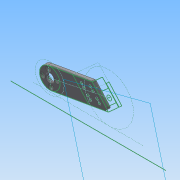
# Autodesk Inventor part: Motor Mount
Saved by Autodesk Inventor 2014 SP2 (Build 180246200, 246)
## iProperties
Created: 2014-05-16
Part Number: Motor Mount
Material: Generic
Document SubType Name: Modeling
Designer: dliu
Density: 1 g/cm^3
Appearance: Default
Author: dliu
Autodesk Inventor part; units mm, degrees
ref_plane "YZ Plane" through (0, 0, 0) normal (1, 0, 0) x (0, 1, 0)
ref_plane "XZ Plane" through (0, 0, 0) normal (0, 1, 0) x (-1, 0, 0)
ref_plane "XY Plane" through (0, 0, 0) normal (0, 0, 1) x (1, 0, 0)
derived "MountSketch.ipt"
sketch "Axle Centers" plane through (0, 0, 0) normal (0, 0, 1) x (1, 0, 0)
  circle A0 centre (-15.5434, 65.9421) radius 41.5 construction
  circle A1 centre (-116.5338, 44.7621) radius 3.5 construction
  circle A2 centre (-116.5338, 44.7621) radius 24.5 construction
  line L0 (-116.5338, 44.7621) -> (-15.5434, 65.9421) construction
  line L1 (81.0038, 7.2633) -> (-183.1725, 7.2633)
  line L2 (43.2643, 24.4421) -> (-145.433, 24.4421) construction
  line L3 (-29.6645, 68.1495) -> (-16.8525, 79.6855)
  line L4 (-16.2626, 80.2166) -> (-3.0043, 65.4918)
  line L5 (-3.0043, 65.4918) -> (-3.5942, 64.9607) construction
  line L6 (-16.4062, 53.4247) -> (-29.6645, 68.1495)
  line L7 (-15.7926, 89.1846) -> (-20.5116, 84.9356)
  line L8 (-38.6325, 68.6195) -> (-16.8762, 44.4567)
  line L9 (-16.8762, 44.4567) -> (0.6548, 60.2417)
  line L10 (5.9636, 65.0218) -> (-15.7926, 89.1846)
  circle A3 centre (-15.5434, 65.9421) radius 3.9688
  line L11 (-44.5107, 75.148) -> (-119.554, 61.9995)
  line L12 (-113.5136, 27.5247) -> (-16.8762, 44.4567)
  line L13 (-119.554, 61.9995) -> (-113.5136, 27.5247) construction
  circle A4 centre (-116.5338, 44.7621) radius 17.5
  line L14 (-38.6325, 68.6195) -> (-44.5107, 75.148)
  line L15 (-77.5896, 69.3522) -> (-49.955, 38.6609)
  line L16 (-62.5555, 64.1664) -> (-58.3065, 59.4475) construction
  circle A5 centre (-62.5555, 64.1664) radius 2.3813 construction
  circle A6 centre (-58.3065, 59.4475) radius 2.3813 construction
  line L17 (-47.3816, 66.8251) -> (-43.1326, 62.1061) construction
  circle A7 centre (-43.1326, 62.1061) radius 2.3813 construction
  circle A8 centre (-47.3816, 66.8251) radius 2.3813 construction
  line L18 (-16.2626, 80.2166) -> (-16.1699, 80.1136)
  circle A9 centre (-36.1592, 54.3614) radius 2.3813 construction
  line L19 (-36.1592, 54.3614) -> (-31.9103, 49.6425) construction
  circle A10 centre (-31.9103, 49.6425) radius 2.3813 construction
  circle A11 centre (-51.3332, 51.7028) radius 2.3813 construction
  line L20 (-51.3332, 51.7028) -> (-47.0842, 46.9838) construction
  circle A12 centre (-47.0842, 46.9838) radius 2.3813 construction
  line L21 (-77.5896, 69.3522) -> (-33.5995, 108.961) construction
  line L22 (-33.5995, 108.961) -> (-15.7926, 89.1846) construction
  line L23 (-44.5107, 75.148) -> (-26.9798, 90.9329)
  line L24 (-26.9798, 90.9329) -> (0.6548, 60.2417)
  line L25 (-20.5116, 84.9356) -> (-38.6325, 68.6195) construction
  line L26 (-20.5116, 84.9356) -> (1.2447, 60.7728)
  line L27 (-3.5942, 64.9607) -> (-16.4062, 53.4247)
  line L28 (-16.8525, 79.6855) -> (-16.2626, 80.2166) construction
  line L29 (0.6548, 60.2417) -> (1.2447, 60.7728) construction
  line L30 (1.2447, 60.7728) -> (5.9636, 65.0218)
  point P0 (-118.6911, 57.0745)
  point P1 (-128.8462, 42.6048)
  point P2 (-114.3765, 32.4496)
  point P3 (-104.2214, 46.9194)
extrude "Extrusion1" add sketch "Axle Centers" against normal blind 6.35 contours L14 L8 L12 L15 L11 | L15 L12 A4 L11 | A4
hole "Hole2" at (-116.5338, 44.7621, 0) direction (0, 0, -1) diameter 15.24 end through all
hole "Hole3" at (-118.6911, 57.0745, 0) at (-128.8462, 42.6048, 0) at (-114.3765, 32.4496, 0) at (-104.2214, 46.9194, 0) direction (0, 0, -1) diameter 4.4958 end through all countersink diameter 9.398 countersink angle 90 clearance for "Flat Head Machine Screw" size "M4" standard "Ansi Metric M Profile"
sketch "Sketch2" plane through (0, 0, 0) normal (0, 0, 1) x (1, 0, 0)
  circle A0 centre (-43.1326, 62.1061) radius 2.3813 projected
  circle A1 centre (-58.3065, 59.4475) radius 2.3813 projected
  circle A2 centre (-47.0842, 46.9838) radius 2.3813 projected
  circle A3 centre (-31.9103, 49.6425) radius 2.3813 projected
  point P0 (0, 0)
extrude "Attachment Holes" cut sketch "Sketch2" along normal through all both and the other way through all
fillet "Fillet1" radius 3.175 2 edges at (-16.8762, 44.4567, -3.175) (-44.5107, 75.148, -3.175)
pattern_linear "Extra Holes" count 2 spacing 6.35 along (-0.6691306, 0.7431448, 0) of "Attachment Holes"
body "Solid1"
